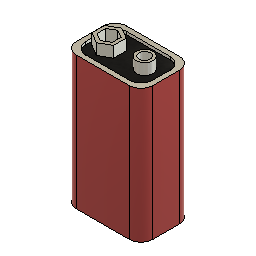
Gecko - Major Product v35 (Autodesk Fusion 360 archive; units mm, degrees)
design "9v Battery"
Autodesk Fusion 360 part; units mm, degrees
sketch "base Sketch" plane through (0, 0, 0) normal (0, 1, 0) x (1, 0, 0)
  line L0 (12.9, -8.5) -> (-12.9, -8.5)
  line L1 (-12.9, -8.5) -> (-12.9, 8.5)
  line L2 (-12.9, 8.5) -> (12.9, 8.5)
  line L3 (12.9, 8.5) -> (12.9, -8.5)
  line L4 (12.9, -8.5) -> (-12.9, 8.5) construction
  line L5 (-12.9, -8.5) -> (12.9, 8.5) construction
  circle A0 centre (5.625, 0) radius 2.775
  circle A1 centre (5.625, 0) radius 1.875
  circle A2 centre (-6.4, -0.0017) radius 2.0246 construction
  line L6 (-6.3962, -4.2517) -> (-2.7175, -2.1234)
  line L7 (-2.7175, -2.1234) -> (-2.7213, 2.1266)
  line L8 (-2.7213, 2.1266) -> (-6.4038, 4.2483)
  line L9 (-6.4038, 4.2483) -> (-10.0825, 2.12)
  line L10 (-10.0825, 2.12) -> (-10.0787, -2.13)
  line L11 (-10.0787, -2.13) -> (-6.3962, -4.2517)
  line L12 (-6.4027, 2.9781) -> (-8.9819, 1.4859)
  line L13 (-8.9819, 1.4859) -> (-8.9793, -1.4939)
  line L14 (-8.9793, -1.4939) -> (-6.3973, -2.9815)
  line L15 (-6.3973, -2.9815) -> (-3.8181, -1.4893)
  line L16 (-3.8181, -1.4893) -> (-3.8207, 1.4905)
  line L17 (-3.8207, 1.4905) -> (-6.4027, 2.9781)
  line L18 (-11.3, -6.9) -> (-11.3, 6.9)
  line L19 (-11.3, 6.9) -> (11.3, 6.9)
  line L20 (11.3, 6.9) -> (11.3, -6.9)
  line L21 (11.3, -6.9) -> (-11.3, -6.9)
  point P0 (-6.4, -0.0017)
  dimension "d1" = 25.8
  dimension "d2" = 17
  dimension "d3" = 5.55
  dimension "d4" = 7.275
  dimension "d5" = -0.9
  dimension "d6" = 6.5
  dimension "d7" = 4.25
  dimension "d8" = -1.1
  dimension "d15" = 1.6
  constraint horizontal L0
  constraint perpendicular L0 L1
  constraint parallel L0 L2
  constraint parallel L1 L3
  constraint coincident L4 origin
  constraint coincident L5 origin
  constraint horizontal origin A0.centre
  constraint coincident P0 A2.centre
  measures "d1" distance of L1.end L2.end
  measures "d2" distance of L0.end L1.end
  measures "d3" diameter of A0
  measures "d4" distance of L3 A0.centre
  measures "d6" distance of L1 P0
  measures "d7" distance of L6.start P0
extrude "Extrude1" add sketch "base Sketch" against normal blind 44 contours L0 L1 L2 L3 | A0 | A1 | L6 L7 L8 L9 L10 L11 | L12 L13 L14 L15 L16 L17 | L18 L19 L20 L21
extrude "Extrude2" add sketch "base Sketch" along normal blind 3.75 contours A0 | L6 L7 L8 L9 L10 L11
extrude "Extrude3" add sketch "base Sketch" along normal blind 1 contours L0 L1 L2 L3
fillet "Fillet1" radius 4 8 edges at (12.9, -21.5, 8.5) (-12.9, -21.5, 8.5) (-12.9, -21.5, -8.5) (12.9, -21.5, -8.5) (11.3, 0.5, 6.9) (-11.3, 0.5, 6.9) (-11.3, 0.5, -6.9) (11.3, 0.5, -6.9)
equation "d4 = 4.5 mm + d3 / 2"
equation "d7 = ( 8.5 / 2 ) * 1 mm"
named bodies: "9V"

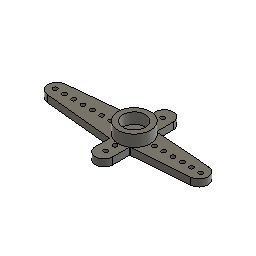
design "Servo Horn - Large"
Autodesk Fusion 360 part; units mm, degrees
sketch "Sketch1" plane through (0, 0, 0) normal (0, 1, 0) x (1, 0, 0)
  circle A0 centre (0, 0) radius 1.125
  circle A1 centre (0, 0) radius 3.5
  line L0 (0, 0) -> (13.95, 0) construction
  line L1 (0, 0) -> (-16.65, 0) construction
  line L2 (0, 0) -> (0, 6.5) construction
  line L3 (0, 0) -> (0, -6.5) construction
  circle A2 centre (0, 6.5) radius 1.9
  circle A3 centre (0, -6.5) radius 1.9
  circle A4 centre (13.95, 0) radius 1.95
  circle A5 centre (-16.65, 0) radius 1.95
  line L4 (14.0995, 1.9443) -> (1.9961, 2.875)
  line L5 (14.0995, -1.9443) -> (1.9961, -2.875)
  line L6 (-16.8396, 1.9408) -> (-1.9, 3.4)
  line L7 (1.9, 6.5) -> (1.9, 2.9394)
  line L8 (-1.9, 6.5) -> (-1.9, 3.4)
  line L9 (-1.9, -3.4) -> (-1.9, -6.5)
  line L10 (1.9, -2.9394) -> (1.9, -6.5)
  circle A6 centre (0, 0) radius 2.4
  circle A7 centre (8.35, 0) radius 0.45
  circle A8 centre (10.35, 0) radius 0.45
  circle A9 centre (12.35, 0) radius 0.45
  circle A10 centre (0, -6.15) radius 0.45
  circle A11 centre (0, -4.15) radius 0.45
  circle A12 centre (14.35, 0) radius 0.45
  circle A13 centre (6.35, 0) radius 0.45
  circle A14 centre (4.35, 0) radius 0.45
  line L11 (-16.8396, -1.9408) -> (-1.9, -3.4)
  circle A15 centre (0, 6.15) radius 0.45
  circle A16 centre (0, 4.15) radius 0.45
  circle A17 centre (-17.05, 0) radius 0.45
  circle A18 centre (-15.05, 0) radius 0.45
  circle A19 centre (-13.05, 0) radius 0.45
  circle A20 centre (-11.05, 0) radius 0.45
  circle A21 centre (-9.05, 0) radius 0.45
  circle A22 centre (-7.05, 0) radius 0.45
  circle A23 centre (-5.05, 0) radius 0.45
  circle A24 centre (0, 0) radius 2.3
  line L12 (1.9961, -2.875) -> (15.9, -2.875) construction
  line L13 (15.9, -2.875) -> (15.9, 0) construction
  line L14 (-1.9, -3.4) -> (-18.6, -3.4) construction
  line L15 (-18.6, -3.4) -> (-18.6, 0) construction
  line L16 (3.0895, -8.4) -> (-2.3757, -8.4) construction
  line L17 (0, -6.6) -> (0, -8.4) construction
  line L18 (-1.67, 8.4) -> (1.1298, 8.4) construction
  line L19 (0, 8.4) -> (0, 6.6) construction
  dimension "d1" = 3.8
  dimension "d2" = 3.9
  dimension "d3" = 3.8
  dimension "d4" = 3.9
  dimension "d6" = 16.65
  dimension "d9" = 7
  dimension "d10" = 2.25
  dimension "d11" = 2.875
  dimension "d12" = 2.875
  dimension "d22" = 0.9
  dimension "d23" = 0.9
  dimension "d24" = 0.9
  dimension "d25" = 0.9
  dimension "d29" = 0.35
  dimension "d30" = 0.9
  dimension "d33" = 0.9
  dimension "d34" = 2
  dimension "d35" = 2
  dimension "d36" = 2
  dimension "d41" = 0.4
  dimension "d42" = 2
  dimension "d43" = 2
  dimension "d44" = 0.9
  dimension "d45" = 0.9
  dimension "d48" = 3.4
  dimension "d49" = 3.4
  dimension "d51" = 3.1
  dimension "d52" = 3.1
  dimension "d55" = 0.9
  dimension "d56" = 0.9
  dimension "d57" = 0.9
  dimension "d58" = 0.9
  dimension "d59" = 0.9
  dimension "d60" = 0.9
  dimension "d61" = 0.9
  dimension "d62" = 0.9
  dimension "d63" = 0.9
  dimension "d64" = 0.4
  dimension "d65" = 2
  dimension "d66" = 2
  dimension "d67" = 2
  dimension "d68" = 2
  dimension "d69" = 2
  dimension "d70" = 2
  dimension "d72" = 4.6
  dimension "d73" = 1.1
  dimension "d76" = 4.8
  dimension "d81" = 13.9039
  dimension "d83" = 14
  dimension "d84" = 16.7
  dimension "d85" = 2
  dimension "d86" = 2
  dimension "d87" = 1.8
  dimension "d88" = 0.35
  dimension "d89" = 1.8
  dimension "d90" = 5
  dimension "d91" = 5.525
  constraint coincident A0.centre A1.centre
  constraint horizontal L0
  constraint parallel L0 L1
  constraint perpendicular L0 L2
  constraint vertical L3
  constraint coincident L2.end A2.centre
  constraint coincident L3.end A3.centre
  constraint coincident L0.end A4.centre
  constraint coincident L1.end A5.centre
  constraint coincident A1 L4.end
  constraint coincident A4 L4.start
  constraint coincident A4 L5.start
  constraint coincident A1 L5.end
  constraint coincident A5 L6.start
  constraint coincident A5 L11.start
  constraint tangent A4 L4
  constraint tangent A4 L5
  constraint tangent A5 L11
  constraint tangent A5 L6
  constraint coincident A2 L7.start
  constraint parallel L2 L7
  constraint tangent A2 L7
  constraint coincident A1 L7.end
  constraint coincident A2 L8.start
  constraint coincident A3 L9.end
  constraint coincident A3 L10.end
  constraint tangent A3 L10
  constraint tangent A3 L9
  constraint tangent A2 L8
  constraint parallel L2 L8
  constraint parallel L3 L10
  constraint parallel L3 L9
  constraint coincident A1 L10.start
  constraint coincident L0 A7.centre
  constraint coincident L0 A8.centre
  constraint coincident L0 A9.centre
  constraint coincident L3 A10.centre
  constraint coincident L3 A11.centre
  constraint coincident L0 A12.centre
  constraint coincident L0 A13.centre
  constraint coincident L0 A14.centre
  constraint coincident L2 A16.centre
  constraint vertical A15.centre A16.centre
  constraint horizontal L1.end A17.centre
  constraint coincident L1 A18.centre
  constraint coincident L1 A19.centre
  constraint coincident L1 A21.centre
  constraint coincident L1 A22.centre
  constraint coincident L1 A23.centre
  constraint concentric A1 A6
  constraint coincident A4 L13.end
  constraint tangent A4 L13
  constraint vertical L13
  constraint horizontal L12
  constraint perpendicular L9 L14
  constraint coincident A5 L15.end
  constraint perpendicular L14 L15
  constraint tangent A5 L15
  constraint horizontal L16
  constraint tangent A3 L16
  constraint coincident A10 L17.start
  constraint coincident L16 L17.end
  constraint coincident A3 L17.end
  constraint perpendicular L16 L17
  constraint horizontal L18
  constraint tangent A2 L18
  constraint coincident A2 L19.start
  constraint coincident A15 L19.end
  constraint perpendicular L18 L19
  measures "d1" diameter of A2
  measures "d2" diameter of A4
  measures "d3" diameter of A3
  measures "d4" diameter of A5
  measures "d6" distance of A0.centre L1.end
  measures "d9" diameter of A1
  measures "d10" diameter of A0
  measures "d11" distance of L0 L5.end
  measures "d12" distance of L0 L4.end
  measures "d22" diameter of A7
  measures "d23" diameter of A8
  measures "d24" diameter of A9
  measures "d25" diameter of A10
  measures "d29" distance of L3.end A10.centre
  measures "d30" diameter of A11
  measures "d33" diameter of A12
  measures "d34" distance of A9.centre A12.centre
  measures "d35" distance of A8.centre A9.centre
  measures "d36" distance of A7.centre A8.centre
  measures "d41" distance of L0.end A12.centre
  measures "d42" distance of A7.centre A13.centre
  measures "d43" distance of A13.centre A14.centre
  measures "d44" diameter of A13
  measures "d45" diameter of A14
  measures "d48" distance of L1 L9.start
  measures "d49" distance of L1 L6.end
  measures "d51" vertical distance of L3.end L9.start
  measures "d52" vertical distance of L2.end L6.end
  measures "d55" diameter of A16
  measures "d56" diameter of A15
  measures "d57" diameter of A17
  measures "d58" diameter of A18
  measures "d59" diameter of A19
  measures "d60" diameter of A20
  measures "d61" diameter of A21
  measures "d62" diameter of A22
  measures "d63" diameter of A23
  measures "d64" distance of L1.end A17.centre
  measures "d65" distance of A17.centre A18.centre
  measures "d66" distance of A18.centre A19.centre
  measures "d67" distance of A19.centre A20.centre
  measures "d68" distance of A20.centre A21.centre
  measures "d69" distance of A21.centre A22.centre
  measures "d70" distance of A22.centre A23.centre
  measures "d72" diameter of A24
  measures "d73" distance of A1 A6
  measures "d76" diameter of A6
  measures "d81" distance of L5.end L12.end
  measures "d83" distance of L10 L13
  measures "d84" distance of L9.start L14.end
  measures "d85" distance of A10.centre A11.centre
  measures "d86" distance of A15.centre A16.centre
  measures "d87" distance of L17.start L17.end
  measures "d88" distance of L2.end A15.centre
  measures "d89" distance of L19.start L19.end
  measures "d90" distance of L9.start L16
  measures "d91" distance of L5.end L16
extrude "Extrude2" add sketch "Sketch1" along normal blind 4 contours A1 | A6 | A24
extrude "Extrude3" add sketch "Sketch1" along normal blind 1.5 contours A1 A4 L4 L5 A9 | A1 A2 A3 A5 L6 L7 L8 L9 L10 L11 A18 | A4 A9 | A2 | A3 | A5 A18 picked at (13.1485, 0.7143) picked at (-15.8899, -0.7443)
extrude "Extrude4" cut sketch "Sketch1" along normal blind 1 contours A24
extrude "Extrude5" cut sketch "Sketch1" against normal blind 2.35 from surface at 4 contours A6 | A24
equation "d3 = d1"
equation "d6 = 18.6 mm - d4 / 2"
equation "d11 = ( 5.75 / 2 ) * 1 mm"
equation "d12 = d11"
equation "d22 = smallHoles"
equation "d23 = smallHoles"
equation "d24 = smallHoles"
equation "d25 = smallHoles"
equation "d29 = 1.8 mm - d3 / 2 + d25 / 2"
equation "d30 = smallHoles"
equation "d33 = smallHoles"
equation "d34 = 2.9 mm - d33"
equation "d35 = d34"
equation "d36 = d34"
equation "d41 = d2 / 2 - ( 1.1 mm + d33 / 2 )"
equation "d42 = d34"
equation "d43 = d34"
equation "d44 = smallHoles"
equation "d45 = smallHoles"
equation "d51 = 5 mm - d3 / 2"
equation "d52 = 5 mm - d1 / 2"
equation "d55 = smallHoles"
equation "d56 = smallHoles"
equation "d57 = smallHoles"
equation "d58 = smallHoles"
equation "d59 = smallHoles"
equation "d60 = smallHoles"
equation "d61 = smallHoles"
equation "d62 = smallHoles"
equation "d63 = smallHoles"
equation "d64 = d4 / 2 - ( 1.1 mm + d57 / 2 )"
equation "d65 = 2.9 mm - d57"
equation "d66 = d65"
equation "d67 = d65"
equation "d68 = d65"
equation "d69 = d65"
equation "d70 = d65"
equation "smallHoles = 0.9 mm"
equation "d85 = 2.9 mm - smallHoles"
equation "d86 = 2.9 mm - smallHoles"
equation "d88 = 1.8 mm - d1 / 2 + d56 / 2"

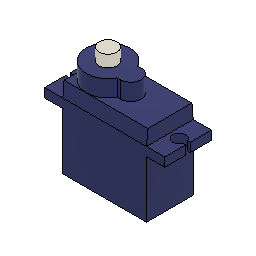
design "TowerPro SG90 Servo Motor - NOAH LOBBE v4"
Autodesk Fusion 360 part; units mm, degrees
sketch "Base" plane through (0, 0, 0) normal (0, 1, 0) x (1, 0, 0)
  line L0 (0, 0) -> (32.25, 0)
  line L1 (32.25, 0) -> (32.25, 12.5)
  line L2 (32.25, 12.5) -> (0, 12.5)
  line L3 (0, 12.5) -> (0, 0)
  line L4 (4.9, 0) -> (4.9, 12.5)
  line L5 (27.35, 0) -> (27.35, 12.5)
  line L6 (4.9, 6.25) -> (10.775, 6.25)
  circle A0 centre (10.775, 6.25) radius 5.875
  circle A1 centre (2.4, 6.25) radius 1.75
  circle A2 centre (29.85, 6.25) radius 1.75
  circle A3 centre (16.9, 6.25) radius 2.75
  line L7 (29.85, 8) -> (32.25, 8)
  line L8 (29.85, 8) -> (29.85, 4.5) construction
  line L9 (29.85, 4.5) -> (32.25, 4.5)
  line L10 (2.4, 8) -> (2.4, 4.5) construction
  line L11 (2.4, 8) -> (0, 8)
  line L12 (2.4, 4.5) -> (0, 4.5)
  line L13 (16.9, 9) -> (16.9, 3.5) construction
  line L14 (16.9, 9) -> (15.1216, 9)
  line L15 (16.9, 3.5) -> (15.1297, 3.5)
  circle A4 centre (10.775, 6.25) radius 2.4
  line L16 (29.85, 6.25) -> (32.4785, 6.25) construction
  line L17 (32.25, 6.85) -> (29.85, 6.85)
  line L18 (32.25, 5.65) -> (29.85, 5.65)
  line L19 (2.4, 6.25) -> (0, 6.25) construction
  line L20 (-1, 5.65) -> (3, 5.65)
  line L21 (-1, 6.85) -> (3, 6.85)
  dimension "d1" = 12.5
  dimension "d2" = 32.25
  dimension "d5" = 4.9
  dimension "d6" = 4.9
  dimension "d7" = 5.875
  dimension "d8" = 11.75
  dimension "d9" = 3.5
  dimension "d10" = 3.5
  dimension "d11" = 6.25
  dimension "d12" = 6.25
  dimension "d13" = 6.25
  dimension "d14" = 6.25
  dimension "d15" = 2.5
  dimension "d16" = 2.5
  dimension "d17" = 5.5
  dimension "d19" = 22.45
  dimension "d32" = 4.8
  dimension "d49" = 12
  dimension "d50" = 10.45
  dimension "d51" = 0.6
  dimension "d52" = 0.6
  dimension "d53" = 0.6
  dimension "d54" = 0.6
  constraint horizontal L0
  constraint vertical L1
  constraint horizontal L2
  constraint vertical L3
  constraint coincident L0.start L3.end
  constraint coincident L0 L4.start
  constraint coincident L2 L4.end
  constraint perpendicular L2 L4
  constraint coincident L0 L5.start
  constraint coincident L2 L5.end
  constraint perpendicular L2 L5
  constraint midpoint L4 L6.start
  constraint perpendicular L4 L6
  constraint coincident L6.end A0.centre
  constraint coincident L6.start A0
  constraint coincident A2 L7.start
  constraint coincident L1 L7.end
  constraint tangent A2 L7
  constraint perpendicular L1 L7
  constraint coincident A2 L8.end
  constraint perpendicular L7 L8
  constraint coincident L1 L9.end
  constraint tangent A2 L9
  constraint coincident A1 L10.start
  constraint coincident A1 L10.end
  constraint vertical L10
  constraint coincident L3 L11.end
  constraint tangent A1 L11
  constraint perpendicular L3 L11
  constraint coincident L3 L12.end
  constraint tangent A1 L12
  constraint horizontal L6.end A3.centre
  constraint coincident A3 L13.start
  constraint coincident A3 L13.end
  constraint vertical L13
  constraint tangent A3 L14
  constraint perpendicular L13 L14
  constraint tangent A3 L15
  constraint concentric A0 A4
  constraint coincident A2.centre L16.start
  constraint perpendicular L1 L16
  constraint horizontal L17
  constraint coincident L1 L17.start
  constraint coincident L8 L17.end
  constraint horizontal L18
  constraint coincident L1 L18.start
  constraint coincident L8 L18.end
  constraint coincident A1.centre L19.start
  constraint perpendicular L3 L19
  constraint coincident L3 L19.end
  constraint perpendicular L10 L20
  constraint horizontal L21
  measures "d1" distance of L0 L2
  measures "d2" distance of L1 L3
  measures "d5" distance of L3 L4
  measures "d6" distance of L1 L5
  measures "d7" distance of L6.start L6.end
  measures "d8" diameter of A0
  measures "d9" diameter of A2
  measures "d10" diameter of A1
  measures "d11" distance of L2 A2.centre
  measures "d12" distance of L0 A2.centre
  measures "d13" distance of L2 A1.centre
  measures "d14" distance of L0 A1.centre
  measures "d15" distance of L4 A1.centre
  measures "d16" distance of L5 A2.centre
  measures "d17" diameter of A3
  measures "d19" distance of L4 L5
  measures "d32" diameter of A4
  measures "d49" distance of L4 A3.centre
  measures "d50" distance of L5 A3.centre
  measures "d51" distance of L16 L17
  measures "d52" distance of L16 L18
  measures "d53" distance of L19 L21
  measures "d54" distance of L19 L20
extrude "Extrude3" add sketch "Base" along normal blind 4 contours A0 A3 | L0 L2 L4 L5 | A0 A3 L14 | A0 A3 L15 | A0 A3 | A0 A3 | A4 makes body 1
extrude "Extrude1" add sketch "Base" against normal blind 17.6 separate body contours A0 A3 | L0 L2 L4 L5 | A0 A3 L14 | A0 A3 L15 | A0 A3 | A0 A3 | A4 makes body 2
extrude "Extrude2" add sketch "Base" against normal blind 2.4 contours L0 L2 L3 L4 A1 L11 L12 | L3 A1 L12 L20 | L0 L1 L2 L5 A2 L7 L9 | L3 A1 L11 L21 | L1 A2 L9 L18 | L1 A2 L7 L17 bodies 2
extrude "Extrude4" add sketch "Base" along normal blind 4.5 from surface at 4 contours A0 A3 | A0 A3 L14 | A0 A3 L15 | A0 A3 | A0 A3 | A4 bodies 1
draft "Draft1" angle -4.75 neutral plane through (0, 0, 0) pull (0, -1, 0) 2 faces at (12.3833, 1.3333, 0) (19.8667, 2.6667, -12.5) on bodies 1
extrude "Extrude5" add sketch "Base" along normal blind 3.2 from surface at 8.5 contours A4 bodies 1
combine "Combine1" operation add target body 1 tool bodies 2
sketch "Wires" plane through (0, -17.6, 0) normal (0, -1, 0) x (1, 0, 0)
  line L0 (5, -8.05) -> (5, -4.45)
  line L1 (5, -4.45) -> (6.25, -4.45)
  line L2 (6.25, -4.45) -> (6.25, -8.05)
  line L3 (6.25, -8.05) -> (5, -8.05)
  line L4 (5, -6.85) -> (6.25, -6.85)
  line L5 (5, -5.65) -> (6.25, -5.65)
  line L6 (27.35, 0) -> (4.9, 0)
  line L7 (4.9, 0) -> (4.9, -12.5)
  line L8 (4.9, -12.5) -> (27.35, -12.5)
  line L9 (27.35, -12.5) -> (27.35, 0)
  dimension "d38" = 3.6
  dimension "d39" = 1.25
  dimension "d40" = 1.2
  dimension "d41" = 1.2
  dimension "d42" = 1.2
  dimension "d56" = 4.45
  dimension "d57" = 0.1
  dimension "d58" = 4.45
  constraint coincident L0 L4.start
  constraint coincident L2 L4.end
  constraint perpendicular L2 L4
  constraint coincident L0 L5.start
  constraint coincident L2 L5.end
  constraint perpendicular L2 L5
  measures "d38" distance of L1 L3
  measures "d39" distance of L0 L2
  measures "d40" distance of L3 L4
  measures "d41" distance of L1 L5
  measures "d42" distance of L4 L5
  measures "d56" distance of L1 L6
  measures "d57" distance of L0 L7
  measures "d58" distance of L3 L8
extrude "Extrude6" add sketch "Wires" along normal blind 3 separate body contours L0 L2 L3 L4 makes body 3
extrude "Extrude7" add sketch "Wires" along normal blind 3 separate body contours L0 L2 L4 L5 makes body 4
extrude "Extrude8" add sketch "Wires" along normal blind 3 separate body contours L0 L1 L2 L5 makes body 5
ref_plane "WorkPlane1" through (10.775, 11.7, -6.25) normal (0, 1, 0) x (0, 0, 1)
sketch "Horn" plane through (10.775, 11.7, -6.25) normal (0, 1, 0) x (1, 0, 0) in component "Horn"
  circle A0 centre (0, 0) radius 2.4
  circle A1 centre (0, 0) radius 3.5
  circle A2 centre (13.9, 0) radius 2
  line L0 (0.3777, 3.4796) -> (14.1158, 1.9883)
  line L1 (0.3777, -3.4796) -> (14.1158, -1.9883)
  circle A3 centre (13.9, 0) radius 0.4
  circle A4 centre (0, 0) radius 1.25
  dimension "d63" = 7
  dimension "d65" = 4
  dimension "d66" = 13.9
  dimension "d67" = 1.1
  dimension "d68" = 4.8
  dimension "d69" = 1.6
  dimension "d70" = 0.8
  dimension "d75" = 2.5
  constraint coincident A0.centre A1.centre
  constraint coincident A1 L0.start
  constraint coincident A2 L0.end
  constraint horizontal A0.centre A2.centre
  constraint tangent A2 L0
  constraint tangent A1 L0
  constraint coincident A1 L1.start
  constraint coincident A2 L1.end
  constraint tangent A1 L1
  constraint tangent A2 L1
  constraint concentric A2 A3
  constraint concentric A0 A4
  measures "d63" diameter of A1
  measures "d65" diameter of A2
  measures "d66" distance of A0.centre A2.centre
  measures "d67" distance of A0 A1
  measures "d68" diameter of A0
  measures "d69" distance of A2 A3
  measures "d70" diameter of A3
  measures "d75" diameter of A4
extrude "Extrude1'" add sketch "Horn" against normal blind 1.3 separate body contours A1 A2 L0 L1 | A2 makes body 6 in component "Horn"
extrude "Extrude2'" add sketch "Horn" against normal blind 3.9 contours A1 bodies 6 in component "Horn"
extrude "Extrude3'" add sketch "Horn" against normal blind 1 from surface at -1 contours A0 bodies 6 in component "Horn"
copy_body "Body->Comp1" bodies 1 removing the originals makes body 7 in component "Servo"
copy_body "Body->Comp2" bodies 3 removing the originals makes body 8 in component "Ground Wire"
copy_body "Body->Comp3" bodies 4 removing the originals makes body 9 in component "Power Wire"
copy_body "Body->Comp4" bodies 5 removing the originals makes body 10 in component "Signal Wire"
component "Servo" placed x (1, 0, 0) y (0, 1, 0) z (0, 0, 1) at (0, 0, 0)
component "Ground Wire" placed x (1, 0, 0) y (0, 1, 0) z (0, 0, 1) at (0, 0, 0)
component "Power Wire" placed x (1, 0, 0) y (0, 1, 0) z (0, 0, 1) at (0, 0, 0)
component "Signal Wire" placed x (1, 0, 0) y (0, 1, 0) z (0, 0, 1) at (0, 0, 0)
equation "d7 = ( 11.75 / 2 ) * 1 mm"
equation "d10 = d9"
equation "d11 = ( d1 / 2 )"
equation "d13 = d1 / 2"
equation "d21 = -( 24 mm - ( 2.4 mm + 4 mm ) )"
equation "d49 = 14.75 mm - ( d17 / 2 )"
equation "d51 = ( 1.2 / 2 ) * 1 mm"
equation "d52 = d51"
equation "d53 = ( 1.2 / 2 ) * 1 mm"
equation "d54 = d53"
equation "d56 = ( d1 - d38 ) / 2"
equation "d66 = 19.4 mm - ( ( d63 / 2 ) + ( d65 / 2 ) )"
named bodies: "Servo", "Ground Wire", "Power Wire", "Signal Wire", "Horn"

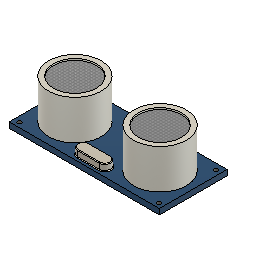
design "Ultrasonic Sensor - NOAH LOBBE v1"
Autodesk Fusion 360 part; units mm, degrees
sketch "Base" plane through (0, 0, 0) normal (0, 1, 0) x (1, 0, 0)
  line L0 (0, 0) -> (45.7, 0)
  line L1 (45.7, 0) -> (45.7, -20.6)
  line L2 (45.7, -20.6) -> (0, -20.6)
  line L3 (0, -20.6) -> (0, 0)
  circle A0 centre (9.9, -10.5) radius 8
  circle A1 centre (35.8, -10.5) radius 8
  circle A2 centre (1.7, -1.8) radius 0.6
  circle A3 centre (1.7, -19.2) radius 0.6
  circle A4 centre (44.2, -19.15) radius 0.6
  circle A5 centre (44.2, -1.8) radius 0.6
  line L4 (18, 0) -> (18, 6)
  line L5 (18, 6) -> (28, 6)
  line L6 (28, 6) -> (28, 0)
  line L7 (18, 0) -> (18, -3)
  line L8 (18, -3) -> (28, -3)
  line L9 (28, 0) -> (28, -3)
  circle A6 centre (9.9, -10.5) radius 6.5
  circle A7 centre (35.8, -10.5) radius 6.5
  line L10 (19.85, -19.6) -> (26.35, -19.6)
  arc A8 (26.35, -19.6) -> (26.35, -16.1) centre (26.35, -17.85) ccw
  line L11 (26.35, -16.1) -> (19.85, -16.1)
  arc A9 (19.85, -16.1) -> (19.85, -19.6) centre (19.85, -17.85) ccw
  line L12 (18.1, -17.85) -> (28.1, -17.85) construction
  line L13 (20, 6) -> (20, -3)
  line L14 (26, 6) -> (26, -3)
  line L15 (24, 6) -> (24, -3)
  line L16 (22, 6) -> (22, -3)
  line L17 (18.7, 6) -> (18.7, -2.1)
  line L18 (19.3, -2.1) -> (19.3, 6)
  line L19 (20.7, 6) -> (20.7, -2.1)
  line L20 (21.3, -2.1) -> (21.3, 6)
  line L21 (22.7, 6) -> (22.7, -2.1)
  line L22 (23.3, -2.1) -> (23.3, 6)
  line L23 (24.7, -2.1) -> (24.7, 6)
  line L24 (25.3, 6) -> (25.3, -2.1)
  line L25 (27.3, -2.1) -> (27.3, 6)
  line L26 (26.7, 6) -> (26.7, -2.1)
  line L27 (17.85, -2.1) -> (27.85, -2.1)
  line L28 (18, -0.1) -> (28, -0.1)
  dimension "d1" = 20.6
  dimension "d2" = 45.7
  dimension "d3" = 9.9
  dimension "d4" = 16
  dimension "d5" = 10.5
  dimension "d6" = 16
  dimension "d7" = 10.5
  dimension "d8" = 9.9
  dimension "d9" = 10.1
  dimension "d10" = 1.2
  dimension "d11" = 1.8
  dimension "d12" = 1.7
  dimension "d13" = 10.1
  dimension "d14" = 1.2
  dimension "d15" = 1.2
  dimension "d16" = 1.2
  dimension "d17" = 1.45
  dimension "d20" = 1.4
  dimension "d21" = 1.5
  dimension "d22" = 1.8
  dimension "d23" = 6
  dimension "d24" = 10
  dimension "d25" = 18
  dimension "d26" = 17.7
  dimension "d35" = 3
  dimension "d36" = -1.5
  dimension "d37" = -1.5
  dimension "d43" = 10
  dimension "d44" = 3.5
  dimension "d45" = 1
  dimension "d49" = 2
  dimension "d50" = 2
  dimension "d51" = 2
  dimension "d52" = 2
  dimension "d53" = 2
  dimension "d59" = 0.6
  dimension "d60" = 0.6
  dimension "d61" = 0.6
  dimension "d62" = 0.6
  dimension "d63" = 0.6
  dimension "d64" = 0.7
  dimension "d65" = 0.7
  dimension "d66" = 0.7
  dimension "d67" = 0.7
  dimension "d68" = 0.7
  dimension "d69" = 0.7
  dimension "d70" = 0.7
  dimension "d73" = 2.1
  dimension "d74" = 0.1
  dimension "d75" = 17.35
  dimension "d76" = 42.5
  dimension "d77" = 18.1
  dimension "d78" = 17.6
  constraint horizontal L0
  constraint vertical L1
  constraint horizontal L2
  constraint vertical L3
  constraint coincident L0.start L3.end
  constraint coincident L0 L4.start
  constraint perpendicular L0 L4
  constraint perpendicular L4 L5
  constraint coincident L0 L6.end
  constraint perpendicular L0 L6
  constraint perpendicular L0 L7
  constraint perpendicular L4 L8
  constraint perpendicular L8 L9
  constraint tangent L10 A8
  constraint tangent A8 L11
  constraint parallel L10 L11
  constraint tangent L11 A9
  constraint tangent L10 A9
  constraint midpoint A9 L12.start
  constraint midpoint A8 L12.end
  constraint coincident L5 L13.start
  constraint coincident L8 L13.end
  constraint perpendicular L8 L13
  constraint coincident L5 L14.start
  constraint coincident L8 L14.end
  constraint perpendicular L8 L14
  constraint coincident L5 L15.start
  constraint coincident L8 L15.end
  constraint perpendicular L5 L15
  constraint coincident L5 L16.start
  constraint coincident L8 L16.end
  constraint perpendicular L8 L16
  constraint coincident L5 L17.start
  constraint perpendicular L0 L17
  constraint coincident L5 L18.end
  constraint perpendicular L5 L18
  constraint coincident L5 L19.start
  constraint perpendicular L0 L19
  constraint coincident L5 L20.end
  constraint perpendicular L0 L20
  constraint coincident L5 L21.start
  constraint perpendicular L0 L21
  constraint coincident L5 L22.end
  constraint perpendicular L5 L22
  constraint coincident L5 L23.end
  constraint perpendicular L5 L23
  constraint coincident L5 L24.start
  constraint perpendicular L0 L24
  constraint coincident L5 L25.end
  constraint perpendicular L5 L25
  constraint coincident L5 L26.start
  constraint perpendicular L0 L26
  constraint coincident L27 L17.end
  constraint coincident L27 L18.start
  constraint coincident L27 L19.end
  constraint coincident L27 L20.start
  constraint coincident L27 L21.end
  constraint coincident L27 L22.start
  constraint coincident L27 L23.start
  constraint coincident L27 L24.end
  constraint coincident L27 L26.end
  constraint coincident L27 L25.start
  constraint coincident L7 L28.start
  constraint coincident L9 L28.end
  constraint perpendicular L9 L28
  constraint vertical A4.centre A5.centre
  constraint vertical A2.centre A3.centre
  measures "d1" distance of L0 L2
  measures "d2" distance of L1 L3
  measures "d3" distance of L3 A0.centre
  measures "d4" diameter of A0
  measures "d5" distance of L0 A0.centre
  measures "d6" diameter of A1
  measures "d7" distance of L0 A1.centre
  measures "d8" distance of L1 A1.centre
  measures "d9" distance of L2 A0.centre
  measures "d10" diameter of A2
  measures "d11" distance of L0 A2.centre
  measures "d12" distance of L3 A2.centre
  measures "d13" distance of L2 A1.centre
  measures "d14" diameter of A5
  measures "d15" diameter of A3
  measures "d16" diameter of A4
  measures "d17" distance of L2 A4.centre
  measures "d20" distance of L2 A3.centre
  measures "d21" distance of L1 A5.centre
  measures "d22" distance of L0 A5.centre
  measures "d23" distance of L0 L5
  measures "d24" distance of L4 L6
  measures "d25" distance of L3 L4
  measures "d26" distance of L1 L6
  measures "d35" distance of L0 L8
  measures "d43" distance of L12.start L12.end
  measures "d44" distance of L10 L11
  measures "d45" distance of L2 L10
  measures "d49" distance of L4 L13
  measures "d50" distance of L13 L16
  measures "d51" distance of L15 L16
  measures "d52" distance of L14 L15
  measures "d53" distance of L6 L14
  measures "d59" distance of L17 L18
  measures "d60" distance of L19 L20
  measures "d61" distance of L21 L22
  measures "d62" distance of L23 L24
  measures "d63" distance of L25 L26
  measures "d64" distance of L6 L25
  measures "d65" distance of L14 L26
  measures "d66" distance of L14 L24
  measures "d67" distance of L15 L22
  measures "d68" distance of L16 L20
  measures "d69" distance of L4 L17
  measures "d70" distance of L13 L18
  measures "d73" distance of L0 L27
  measures "d74" distance of L0 L28
  measures "d75" vertical distance of A4.centre A5.centre
  measures "d76" horizontal distance of A2.centre A5.centre
  measures "d77" distance of L3 L12.start
  measures "d78" distance of L1 L12.end
extrude "Extrude1" add sketch "Base" against normal blind 1.7 contours L0 L1 L2 L3 L7 L8 L9 | L0 L7 L17 L28 | L0 L17 L18 L28 | L7 L17 L27 L28 | L0 L13 L18 L28 | L17 L18 L27 L28 | L7 L8 L13 L27 | L0 L13 L19 L28 | L13 L18 L27 L28 | L0 L9 L25 L28 | L0 L19 L20 L28 | L13 L19 L27 L28 | L8 L13 L16 L27 | L0 L25 L26 L28 | L8 L9 L14 L25 L27 L28 | L0 L16 L20 L28 | L19 L20 L27 L28 | L8 L15 L16 L27 | L0 L14 L26 L28 | L25 L26 L27 L28 | L0 L16 L21 L28 | L16 L20 L27 L28 | L8 L14 L15 L27 | L16 L21 L27 L28 | L0 L14 L24 L28 | L14 L26 L27 L28 | L0 L21 L22 L28 | L15 L22 L27 L28 | L15 L23 L27 L28 | L21 L22 L27 L28 | L0 L23 L24 L28 | L14 L24 L27 L28 | L0 L15 L22 L28 | L0 L15 L23 L28 | L23 L24 L27 L28 | A0 | A1 | A6 | A7 | L10 A8 L11 A9
extrude "Extrude2" add sketch "Base" along normal blind 12 contours A0 | A1
extrude "Extrude6" add 2 faces at (37.8704, 0, 11.1386) (7.8952, 0, 8.3394) along direction (0, 1, 0) blind 11.5
extrude "Extrude7" add sketch "Base" along normal blind 2 contours L10 A8 L11 A9
fillet "Fillet1" radius 0.2 8 edges at (18.1, 2, 17.85) (23.1, 2, 19.6) (28.1, 2, 17.85) (23.1, 2, 16.1) (18.1, 0, 17.85) (23.1, 0, 16.1) (28.1, 0, 17.85) (23.1, 0, 19.6)
extrude "Extrude3" add sketch "Base" against normal blind 3.3 from surface at -1.7 contours L7 L17 L27 L28 | L17 L18 L27 L28 | L7 L8 L13 L27 | L13 L18 L27 L28 | L13 L19 L27 L28 | L8 L13 L16 L27 | L8 L9 L14 L25 L27 L28 | L19 L20 L27 L28 | L8 L15 L16 L27 | L25 L26 L27 L28 | L16 L20 L27 L28 | L8 L14 L15 L27 | L16 L21 L27 L28 | L14 L26 L27 L28 | L15 L22 L27 L28 | L15 L23 L27 L28 | L21 L22 L27 L28 | L14 L24 L27 L28 | L23 L24 L27 L28
extrude "Extrude5" add sketch "Base" against normal blind 0.7 from surface at -5 contours L0 L5 L17 L18 | L0 L17 L18 L28 | L17 L18 L27 L28 | L0 L5 L19 L20 | L0 L19 L20 L28 | L0 L25 L26 L28 | L0 L5 L25 L26 | L19 L20 L27 L28 | L25 L26 L27 L28 | L0 L5 L21 L22 | L0 L21 L22 L28 | L21 L22 L27 L28 | L0 L23 L24 L28 | L0 L5 L23 L24 | L23 L24 L27 L28
equation "d3 = 1.9 mm + ( d4 / 2 )"
equation "d5 = 2.5 mm + ( d4 / 2 )"
equation "d6 = d4"
equation "d7 = 2.5 mm + ( d4 / 2 )"
equation "d8 = 1.9 mm + ( d4 / 2 )"
equation "d11 = 1.2 mm + d10 / 2"
equation "d12 = 1.1 mm + d10 / 2"
equation "d14 = d10"
equation "d15 = d10"
equation "d16 = d10"
equation "d17 = 0.85 mm + d16 / 2"
equation "d20 = 0.8 mm + d15 / 2"
equation "d21 = 0.9 mm + d14 / 2"
equation "d22 = 1.2 mm + d14 / 2"
equation "d40 = 12 mm - 0.5 mm"
equation "d49 = d24 / 5"
equation "d50 = d24 / 5"
equation "d51 = d24 / 5"
equation "d52 = d24 / 5"
equation "d73 = d59 + d35 / 2"
named bodies: "Sensor"
